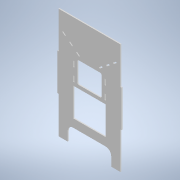
# Autodesk Inventor part: Pared_Frontal
Saved by Autodesk Inventor 2020.1 (Build 241239000, 239)
## iProperties
Created: 2019-12-09
Part Number: Pared_Frontal
Material: Generic
Document SubType Name: Modeling
Designer: Daniel
Density: 1 g/cm^3
Appearance: Default
Author: Daniel
Autodesk Inventor part; units mm, degrees
ref_plane "YZ Plane" through (0, 0, 0) normal (1, 0, 0) x (0, 1, 0)
ref_plane "XZ Plane" through (0, 0, 0) normal (0, 1, 0) x (-1, 0, 0)
ref_plane "XY Plane" through (0, 0, 0) normal (0, 0, 1) x (1, 0, 0)
sketch "Sketch1" plane through (0, 0, 0) normal (0, 0, 1) x (1, 0, 0)
  line L0 (-76.9983, 8.3713) -> (-75.1513, 10.7353) projected
  line L1 (-75.1513, 10.7353) -> (-67.2712, 4.5787) projected
  line L2 (-67.2712, 4.5787) -> (-69.1182, 2.2147) projected
  line L3 (-69.1182, 2.2147) -> (-76.9983, 8.3713) projected
  line L4 (-86.1834, 19.3546) -> (-88.0304, 16.9906) projected
  line L5 (-88.0304, 16.9906) -> (-95.9105, 23.1472) projected
  line L6 (-95.9105, 23.1472) -> (-94.0636, 25.5112) projected
  line L7 (-94.0636, 25.5112) -> (-86.1834, 19.3546) projected
  line L8 (-106.9427, 31.7664) -> (-114.8228, 37.9231) projected
  line L9 (-114.8228, 37.9231) -> (-112.9758, 40.2871) projected
  line L10 (-112.9758, 40.2871) -> (-105.0957, 34.1305) projected
  line L11 (-105.0957, 34.1305) -> (-106.9427, 31.7664) projected
  line L12 (-6.8487, 10.7353) -> (-5.0017, 8.3713) projected
  line L13 (-5.0017, 8.3713) -> (-12.8818, 2.2147) projected
  line L14 (-12.8818, 2.2147) -> (-14.7288, 4.5787) projected
  line L15 (-14.7288, 4.5787) -> (-6.8487, 10.7353) projected
  line L16 (6.0304, 16.9906) -> (4.1834, 19.3546) projected
  line L17 (4.1834, 19.3546) -> (12.0636, 25.5112) projected
  line L18 (12.0636, 25.5112) -> (13.9105, 23.1472) projected
  line L19 (13.9105, 23.1472) -> (6.0304, 16.9906) projected
  line L20 (32.8228, 37.9231) -> (24.9427, 31.7664) projected
  line L21 (24.9427, 31.7664) -> (23.0957, 34.1305) projected
  line L22 (23.0957, 34.1305) -> (30.9758, 40.2871) projected
  line L23 (30.9758, 40.2871) -> (32.8228, 37.9231) projected
  line L24 (-82, 0) -> (-82, -73.9786) construction
  line L25 (-82, -73.9786) -> (-82, -147.5817) construction
  line L26 (-82, -147.5817) -> (-85, -147.5817)
  line L27 (-85, -147.5817) -> (-85, -73.9786)
  line L28 (-85, -73.9786) -> (-85, 0) construction
  line L29 (-85, 0) -> (-82, 0) construction
  line L30 (-85, -73.9786) -> (-82, -73.9786)
  line L31 (3, 0) -> (3, -73.9786) construction
  line L32 (3, -73.9786) -> (3, -147.5817)
  line L33 (3, -147.5817) -> (0, -147.5817)
  line L34 (0, -147.5817) -> (0, -73.9786) construction
  line L35 (0, -73.9786) -> (0, 0) construction
  line L36 (0, 0) -> (3, 0) construction
  line L37 (0, -73.9786) -> (3, -73.9786)
  line L38 (-82, -143.7746) -> (0, -143.7746) construction
  line L39 (0, -143.7746) -> (0, -147.5817)
  line L40 (0, -147.5817) -> (-82, -147.5817)
  line L41 (-82, -147.5817) -> (-82, -143.7746)
  line L42 (-82, -73.9786) -> (0, -73.9786)
  line L43 (-85, -65) -> (-85, -50) projected
  line L44 (-85, -50) -> (-82, -50) projected
  line L45 (-82, -50) -> (-82, -65) projected
  line L46 (-82, -65) -> (-85, -65) projected
  line L47 (3, -50) -> (3, -65) projected
  line L48 (3, -65) -> (0, -65) projected
  line L49 (0, -65) -> (0, -50) projected
  line L50 (0, -50) -> (3, -50) projected
  line L51 (-82, -30) -> (-85, -30) projected
  line L52 (-85, -30) -> (-85, -15) projected
  line L53 (-85, -15) -> (-82, -15) projected
  line L54 (-82, -15) -> (-82, -30) projected
  line L55 (3, -30) -> (0, -30) projected
  line L56 (0, -30) -> (0, -15) projected
  line L57 (0, -15) -> (3, -15) projected
  line L58 (3, -15) -> (3, -30) projected
  line L59 (43, 87) -> (-125, 87) projected
  line L60 (-128, -13) -> (-128, -113) projected
  line L61 (18, -213) -> (43, -213) projected
  line L62 (46, -113) -> (46, -13) projected
  line L63 (-125, -113) -> (-125, -213) projected
  line L64 (43, -213) -> (43, -113) projected
  line L65 (43, -113) -> (46, -113) projected
  line L66 (46, -13) -> (43, -13) projected
  line L67 (43, -13) -> (43, 87) projected
  line L68 (-125, 87) -> (-125, -13) projected
  line L69 (-125, -13) -> (-128, -13) projected
  line L70 (-128, -113) -> (-125, -113) projected
  line L71 (-100, -213) -> (-100, -188) projected
  arc A0 (-85, -173) -> (-100, -188) centre (-85, -188) ccw projected
  line L72 (-85, -173) -> (3, -173) projected
  arc A1 (18, -188) -> (3, -173) centre (3, -188) ccw projected
  line L73 (18, -188) -> (18, -213) projected
  line L74 (-125, -213) -> (-100, -213) projected
  constraints: 38 end point, 10 vertical, 8 horizontal, 1 perpendicular, 13 other
extrude "Extrusion1" add sketch "Sketch1" along normal blind 3
sketch "Sketch2" plane through (0, 0, 3) normal (0, 0, 1) x (1, 0, 0)
  line L0 (-82, -76.3225) -> (-82, -149.9255)
  line L1 (-82, -149.9255) -> (-85, -149.9255)
  line L2 (-85, -149.9255) -> (-85, -76.3225)
  line L3 (-85, -76.3225) -> (-82, -76.3225)
  line L4 (-82, -146.1185) -> (0, -146.1185)
  line L5 (0, -146.1185) -> (0, -149.9255)
  line L6 (0, -149.9255) -> (-82, -149.9255)
  line L7 (-82, -149.9255) -> (-82, -146.1185)
  line L8 (3, -76.3225) -> (3, -149.9255)
  line L9 (3, -149.9255) -> (0, -149.9255)
  line L10 (0, -149.9255) -> (0, -76.3225)
  line L11 (0, -76.3225) -> (3, -76.3225)
  point P0 (0, 0)
  constraints: 24 end point, 6 horizontal, 6 vertical, 10 other
extrude "Extrusion2" cut sketch "Sketch2" against normal blind 10
sketch "Sketch4" plane through (0, 0, 3) normal (0, 0, 1) x (1, 0, 0)
  line L0 (-85, -149.9255) -> (3, -149.9255) projected
  line L1 (-85, -149.9255) -> (3, -149.9255)
  line L2 (3, -149.9255) -> (3, -150.9255)
  line L3 (3, -150.9255) -> (-85, -150.9255)
  line L4 (-85, -150.9255) -> (-85, -149.9255)
  line L5 (3, -73.9786) -> (3, -149.9255) projected
  point P0 (0, 0)
  point P1 (3, -149.9255)
  dimension "d6" = 1
  constraints: 8 end point, 2 parallel, 1 collinear, 1 horizontal, 1 perpendicular
  measures "d6" distance of L1.end L2.end
extrude "Extrusion4" cut sketch "Sketch4" against normal blind 10
sketch "Sketch6" plane through (0, 0, 3) normal (0, 0, 1) x (1, 0, 0)
  line L0 (-100, -213) -> (18, -213)
  line L1 (18, -213) -> (18, -173)
  line L2 (18, -173) -> (-100, -173)
  line L3 (-100, -173) -> (-100, -213)
  line L4 (-125, -113) -> (-125, -213) projected
  line L5 (43, -213) -> (43, -113) projected
  line L6 (-125, -213) -> (43, -213) projected
  point P0 (0, 0)
  dimension "d9" = 25
  dimension "d10" = 25
  dimension "d11" = 40
  constraints: 8 end point, 2 parallel, 1 collinear, 1 horizontal, 1 perpendicular
  measures "d9" distance between parallel lines of L4 L3
  measures "d10" distance between parallel lines of L5 L1
  measures "d11" distance of L0.end L1.end
extrude "Extrusion5" cut sketch "Sketch6" against normal blind 10
fillet "Fillet1" radius 15 2 edges at (-100, -173, 1.5) (18, -173, 1.5)
sketch "Sketch7" plane through (0, 0, 3) normal (0, 0, 1) x (1, 0, 0)
  line L0 (-74, -64.9786) -> (-8, -64.9786)
  line L1 (-8, -64.9786) -> (-8, -6.9786)
  line L2 (-8, -6.9786) -> (-74, -6.9786)
  line L3 (-74, -6.9786) -> (-74, -64.9786)
  line L4 (0, -65) -> (0, -50) projected
  line L5 (-82, -50) -> (-82, -65) projected
  line L6 (-85, -73.9786) -> (3, -73.9786) projected
  dimension "d15" = 8
  dimension "d16" = 8
  dimension "d17" = 9
  dimension "d18" = 58
  constraints: 8 end point, 2 parallel, 1 horizontal, 1 perpendicular
  measures "d15" distance between parallel lines of L1 L4
  measures "d16" distance between parallel lines of L3 L5
  measures "d17" distance between parallel lines of L0 L6
  measures "d18" distance between parallel lines of L0 L2
extrude "Extrusion6" cut sketch "Sketch7" against normal blind 10
fillet "Fillet2" radius 4 4 edges at (-74, -6.9786, 1.5) (-8, -6.9786, 1.5) (-8, -64.9786, 1.5) (-74, -64.9786, 1.5)
body "Solid1"
